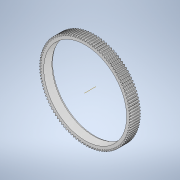
# Autodesk Inventor part: МТ10-3.00.00.01
Saved by Autodesk Inventor 2021 (Build 250183000, 183)
## iProperties
Created: 2022-06-08
Part Number: МТ10-3.00.00.01
Material: Типовые
Document SubType Name: Modeling
Designer: u
Density: 1 g/cm^3
Appearance: По умолчанию
Mass: 620.535 g
Surface Area: 1629.14 cm^2
Volume: 620.535 cm^3
Description: Колесо
Author: u
Title: Колесо
Autodesk Inventor part; units mm, degrees
ref_plane "YZ Plane" through (0, 0, 0) normal (1, 0, 0) x (0, 1, 0)
ref_plane "XZ Plane" through (0, 0, 0) normal (0, 1, 0) x (-1, 0, 0)
ref_plane "XY Plane" through (0, 0, 0) normal (0, 0, 1) x (1, 0, 0)
sketch "Эскиз1" plane through (0, 0, 0) normal (0, 0, 1) x (1, 0, 0)
  circle A0 centre (0, 0) radius 172
  circle A1 centre (0, 0) radius 189.5
  circle A2 centre (0, 0) radius 175.25
  dimension "d0" = 344
  dimension "d1" = 350.5
  dimension "d2" = 379
  constraints: 3 centre point, 3 coincident
  measures "d0" diameter of A0
  measures "d1" diameter of A2
  measures "d2" diameter of A1
extrude "Выдавливание1" add sketch "Эскиз1" along normal blind 40 contours A1 | A2
sketch "Эскиз3" plane through (0, 0, 0) normal (0, 0, -1) x (-1, 0, 0)
  circle A0 centre (0, 0) radius 183
  line L0 (-3.8538, 189.4608) -> (-1.5, 182.9939)
  line L1 (3.8538, 189.4608) -> (1.5, 182.9939)
  circle A1 centre (0, 0) radius 189.5 projected
  line L2 (0, 183) -> (0, 189.5)
  line L3 (-14.6636, 188.9318) -> (-11.9445, 182.6098)
  line L4 (-6.9686, 189.3718) -> (-8.9493, 182.781)
  line L5 (-25.4256, 187.7866) -> (-22.3499, 181.6301)
  line L6 (-17.7682, 188.6652) -> (-19.3695, 181.972)
  line L7 (-36.1046, 186.0288) -> (-32.6825, 180.0579)
  line L8 (-28.5099, 187.3431) -> (-29.7265, 180.5695)
  line L9 (-46.6659, 183.6642) -> (-42.9085, 177.8984)
  line L10 (-39.1586, 185.41) -> (-39.9865, 178.5779)
  line L11 (-57.075, 180.7006) -> (-52.9946, 175.1587)
  line L12 (-49.6796, 182.8721) -> (-50.1161, 176.0039)
  line L13 (-67.2979, 177.1475) -> (-62.9077, 171.8477)
  line L14 (-60.0385, 179.7377) -> (-60.0822, 172.8558)
  line L15 (-77.3012, 173.0167) -> (-72.6157, 167.9761)
  line L16 (-70.2016, 176.017) -> (-69.8524, 169.1439)
  line L17 (-87.0525, 168.3215) -> (-82.0868, 163.5566)
  line L18 (-80.1357, 171.7222) -> (-79.3947, 164.8802)
  line L19 (-96.5198, 163.0772) -> (-91.2902, 158.6036)
  line L20 (-89.8085, 166.8673) -> (-88.678, 160.0788)
  line L21 (-105.6723, 157.3011) -> (-100.1958, 153.1333)
  line L22 (-99.1882, 161.4681) -> (-97.6721, 154.7552)
  line L23 (-114.48, 151.0118) -> (-108.7746, 147.1635)
  line L24 (-108.2445, 155.5422) -> (-106.3476, 148.9268)
  line L25 (-122.9144, 144.23) -> (-116.9986, 140.7136)
  line L26 (-116.9477, 149.109) -> (-114.6762, 142.6127)
  line L27 (-130.9479, 136.9777) -> (-124.841, 133.8048)
  line L28 (-125.2694, 142.1894) -> (-122.6307, 135.8334)
  line L29 (-138.5542, 129.2787) -> (-132.2761, 126.4596)
  line L30 (-133.1825, 134.806) -> (-130.1853, 128.611)
  line L31 (-145.7086, 121.158) -> (-139.2798, 118.7019)
  line L32 (-140.6612, 126.9829) -> (-137.3152, 120.9691)
  line L33 (-152.3877, 112.642) -> (-145.8292, 110.557)
  line L34 (-147.6811, 118.7457) -> (-143.9973, 112.9327)
  line L35 (-158.5698, 103.7587) -> (-151.9029, 102.0514)
  line L36 (-154.2193, 110.1211) -> (-150.2096, 104.5278)
  line L37 (-164.2347, 94.5369) -> (-157.4812, 93.213)
  line L38 (-160.2545, 101.1373) -> (-155.932, 95.7821)
  line L39 (-169.3638, 85.0068) -> (-162.5458, 84.0706)
  line L40 (-165.7669, 91.8236) -> (-161.1458, 86.7239)
  line L41 (-173.9405, 75.1993) -> (-167.0802, 74.6539)
  line L42 (-170.7387, 82.2104) -> (-165.8339, 77.3828)
  line L43 (-177.9499, 65.1466) -> (-171.0696, 64.9938)
  line L44 (-175.1535, 72.329) -> (-169.9812, 67.7894)
  line L45 (-181.3788, 54.8814) -> (-174.501, 55.1216)
  line L46 (-178.9971, 62.2118) -> (-173.574, 57.9748)
  line L47 (-184.2161, 44.4372) -> (-177.3633, 45.0697)
  line L48 (-182.2567, 51.8916) -> (-176.6006, 47.9711)
  line L49 (-186.4526, 33.8481) -> (-179.647, 34.8707)
  line L50 (-184.9219, 41.4021) -> (-179.0512, 37.811)
  line L51 (-188.0808, 23.1485) -> (-181.3447, 24.558)
  line L52 (-186.9839, 30.7776) -> (-180.9178, 27.5275)
  line L53 (-189.0956, 12.3735) -> (-182.4509, 14.1652)
  line L54 (-188.436, 20.0528) -> (-182.1942, 17.1542)
  line L55 (-189.4936, 1.558) -> (-182.9621, 3.7262)
  line L56 (-189.2735, 9.2625) -> (-182.8764, 6.725)
  line L57 (-189.2735, -9.2625) -> (-182.8764, -6.725)
  line L58 (-189.4936, -1.558) -> (-182.9621, -3.7262)
  line L59 (-188.436, -20.0528) -> (-182.1942, -17.1542)
  line L60 (-189.0956, -12.3735) -> (-182.4509, -14.1652)
  line L61 (-186.9839, -30.7776) -> (-180.9178, -27.5275)
  line L62 (-188.0808, -23.1485) -> (-181.3447, -24.558)
  line L63 (-184.9219, -41.4021) -> (-179.0512, -37.811)
  line L64 (-186.4526, -33.8481) -> (-179.647, -34.8707)
  line L65 (-182.2567, -51.8916) -> (-176.6006, -47.9711)
  line L66 (-184.2161, -44.4372) -> (-177.3633, -45.0697)
  line L67 (-178.9971, -62.2118) -> (-173.574, -57.9748)
  line L68 (-181.3788, -54.8814) -> (-174.501, -55.1216)
  line L69 (-175.1535, -72.329) -> (-169.9812, -67.7894)
  line L70 (-177.9499, -65.1466) -> (-171.0696, -64.9938)
  line L71 (-170.7387, -82.2104) -> (-165.8339, -77.3828)
  line L72 (-173.9405, -75.1993) -> (-167.0802, -74.6539)
  line L73 (-165.7669, -91.8236) -> (-161.1458, -86.7239)
  line L74 (-169.3638, -85.0068) -> (-162.5458, -84.0706)
  line L75 (-160.2545, -101.1373) -> (-155.932, -95.7821)
  line L76 (-164.2347, -94.5369) -> (-157.4812, -93.213)
  line L77 (-154.2193, -110.1211) -> (-150.2096, -104.5278)
  line L78 (-158.5698, -103.7587) -> (-151.9029, -102.0514)
  line L79 (-147.6811, -118.7457) -> (-143.9973, -112.9327)
  line L80 (-152.3877, -112.642) -> (-145.8292, -110.557)
  line L81 (-140.6612, -126.9829) -> (-137.3152, -120.9691)
  line L82 (-145.7086, -121.158) -> (-139.2798, -118.7019)
  line L83 (-133.1825, -134.806) -> (-130.1853, -128.611)
  line L84 (-138.5542, -129.2787) -> (-132.2761, -126.4596)
  line L85 (-125.2694, -142.1894) -> (-122.6307, -135.8334)
  line L86 (-130.9479, -136.9777) -> (-124.841, -133.8048)
  line L87 (-116.9477, -149.109) -> (-114.6762, -142.6127)
  line L88 (-122.9144, -144.23) -> (-116.9986, -140.7136)
  line L89 (-108.2445, -155.5422) -> (-106.3476, -148.9268)
  line L90 (-114.48, -151.0118) -> (-108.7746, -147.1635)
  line L91 (-99.1882, -161.4681) -> (-97.6721, -154.7552)
  line L92 (-105.6723, -157.3011) -> (-100.1958, -153.1333)
  line L93 (-89.8085, -166.8673) -> (-88.678, -160.0788)
  line L94 (-96.5198, -163.0772) -> (-91.2902, -158.6036)
  line L95 (-80.1357, -171.7222) -> (-79.3947, -164.8802)
  line L96 (-87.0525, -168.3215) -> (-82.0868, -163.5566)
  line L97 (-70.2016, -176.017) -> (-69.8524, -169.1439)
  line L98 (-77.3012, -173.0167) -> (-72.6157, -167.9761)
  line L99 (-60.0385, -179.7377) -> (-60.0822, -172.8558)
  line L100 (-67.2979, -177.1475) -> (-62.9077, -171.8477)
  line L101 (-49.6796, -182.8721) -> (-50.1161, -176.0039)
  line L102 (-57.075, -180.7006) -> (-52.9946, -175.1587)
  line L103 (-39.1586, -185.41) -> (-39.9865, -178.5779)
  line L104 (-46.6659, -183.6642) -> (-42.9085, -177.8984)
  line L105 (-28.5099, -187.3431) -> (-29.7265, -180.5695)
  line L106 (-36.1046, -186.0288) -> (-32.6825, -180.0579)
  line L107 (-17.7682, -188.6652) -> (-19.3695, -181.972)
  line L108 (-25.4256, -187.7866) -> (-22.3499, -181.6301)
  line L109 (-6.9686, -189.3718) -> (-8.9493, -182.781)
  line L110 (-14.6636, -188.9318) -> (-11.9445, -182.6098)
  line L111 (3.8538, -189.4608) -> (1.5, -182.9939)
  line L112 (-3.8538, -189.4608) -> (-1.5, -182.9939)
  line L113 (14.6636, -188.9318) -> (11.9445, -182.6098)
  line L114 (6.9686, -189.3718) -> (8.9493, -182.781)
  line L115 (25.4256, -187.7866) -> (22.3499, -181.6301)
  line L116 (17.7682, -188.6652) -> (19.3695, -181.972)
  line L117 (36.1046, -186.0288) -> (32.6825, -180.0579)
  line L118 (28.5099, -187.3431) -> (29.7265, -180.5695)
  line L119 (46.6659, -183.6642) -> (42.9085, -177.8984)
  line L120 (39.1586, -185.41) -> (39.9865, -178.5779)
  line L121 (57.075, -180.7006) -> (52.9946, -175.1587)
  line L122 (49.6796, -182.8721) -> (50.1161, -176.0039)
  line L123 (67.2979, -177.1475) -> (62.9077, -171.8477)
  line L124 (60.0385, -179.7377) -> (60.0822, -172.8558)
  line L125 (77.3012, -173.0167) -> (72.6157, -167.9761)
  line L126 (70.2016, -176.017) -> (69.8524, -169.1439)
  line L127 (87.0525, -168.3215) -> (82.0868, -163.5566)
  line L128 (80.1357, -171.7222) -> (79.3947, -164.8802)
  line L129 (96.5198, -163.0772) -> (91.2902, -158.6036)
  line L130 (89.8085, -166.8673) -> (88.678, -160.0788)
  line L131 (105.6723, -157.3011) -> (100.1958, -153.1333)
  line L132 (99.1882, -161.4681) -> (97.6721, -154.7552)
  line L133 (114.48, -151.0118) -> (108.7746, -147.1635)
  line L134 (108.2445, -155.5422) -> (106.3476, -148.9268)
  line L135 (122.9144, -144.23) -> (116.9986, -140.7136)
  line L136 (116.9477, -149.109) -> (114.6762, -142.6127)
  line L137 (130.9479, -136.9777) -> (124.841, -133.8048)
  line L138 (125.2694, -142.1894) -> (122.6307, -135.8334)
  line L139 (138.5542, -129.2787) -> (132.2761, -126.4596)
  line L140 (133.1825, -134.806) -> (130.1853, -128.611)
  line L141 (145.7086, -121.158) -> (139.2798, -118.7019)
  line L142 (140.6612, -126.9829) -> (137.3152, -120.9691)
  line L143 (152.3877, -112.642) -> (145.8292, -110.557)
  line L144 (147.6811, -118.7457) -> (143.9973, -112.9327)
  line L145 (158.5698, -103.7587) -> (151.9029, -102.0514)
  line L146 (154.2193, -110.1211) -> (150.2096, -104.5278)
  line L147 (164.2347, -94.5369) -> (157.4812, -93.213)
  line L148 (160.2545, -101.1373) -> (155.932, -95.7821)
  line L149 (169.3638, -85.0068) -> (162.5458, -84.0706)
  line L150 (165.7669, -91.8236) -> (161.1458, -86.7239)
  line L151 (173.9405, -75.1993) -> (167.0802, -74.6539)
  line L152 (170.7387, -82.2104) -> (165.8339, -77.3828)
  line L153 (177.9499, -65.1466) -> (171.0696, -64.9938)
  line L154 (175.1535, -72.329) -> (169.9812, -67.7894)
  line L155 (181.3788, -54.8814) -> (174.501, -55.1216)
  line L156 (178.9971, -62.2118) -> (173.574, -57.9748)
  line L157 (184.2161, -44.4372) -> (177.3633, -45.0697)
  line L158 (182.2567, -51.8916) -> (176.6006, -47.9711)
  line L159 (186.4526, -33.8481) -> (179.647, -34.8707)
  line L160 (184.9219, -41.4021) -> (179.0512, -37.811)
  line L161 (188.0808, -23.1485) -> (181.3447, -24.558)
  line L162 (186.9839, -30.7776) -> (180.9178, -27.5275)
  line L163 (189.0956, -12.3735) -> (182.4509, -14.1652)
  line L164 (188.436, -20.0528) -> (182.1942, -17.1542)
  line L165 (189.4936, -1.558) -> (182.9621, -3.7262)
  line L166 (189.2735, -9.2625) -> (182.8764, -6.725)
  line L167 (189.2735, 9.2625) -> (182.8764, 6.725)
  line L168 (189.4936, 1.558) -> (182.9621, 3.7262)
  line L169 (188.436, 20.0528) -> (182.1942, 17.1542)
  line L170 (189.0956, 12.3735) -> (182.4509, 14.1652)
  line L171 (186.9839, 30.7776) -> (180.9178, 27.5275)
  line L172 (188.0808, 23.1485) -> (181.3447, 24.558)
  line L173 (184.9219, 41.4021) -> (179.0512, 37.811)
  line L174 (186.4526, 33.8481) -> (179.647, 34.8707)
  line L175 (182.2567, 51.8916) -> (176.6006, 47.9711)
  line L176 (184.2161, 44.4372) -> (177.3633, 45.0697)
  line L177 (178.9971, 62.2118) -> (173.574, 57.9748)
  line L178 (181.3788, 54.8814) -> (174.501, 55.1216)
  line L179 (175.1535, 72.329) -> (169.9812, 67.7894)
  line L180 (177.9499, 65.1466) -> (171.0696, 64.9938)
  line L181 (170.7387, 82.2104) -> (165.8339, 77.3828)
  line L182 (173.9405, 75.1993) -> (167.0802, 74.6539)
  line L183 (165.7669, 91.8236) -> (161.1458, 86.7239)
  line L184 (169.3638, 85.0068) -> (162.5458, 84.0706)
  line L185 (160.2545, 101.1373) -> (155.932, 95.7821)
  line L186 (164.2347, 94.5369) -> (157.4812, 93.213)
  line L187 (154.2193, 110.1211) -> (150.2096, 104.5278)
  line L188 (158.5698, 103.7587) -> (151.9029, 102.0514)
  line L189 (147.6811, 118.7457) -> (143.9973, 112.9327)
  line L190 (152.3877, 112.642) -> (145.8292, 110.557)
  line L191 (140.6612, 126.9829) -> (137.3152, 120.9691)
  line L192 (145.7086, 121.158) -> (139.2798, 118.7019)
  line L193 (133.1825, 134.806) -> (130.1853, 128.611)
  line L194 (138.5542, 129.2787) -> (132.2761, 126.4596)
  line L195 (125.2694, 142.1894) -> (122.6307, 135.8334)
  line L196 (130.9479, 136.9777) -> (124.841, 133.8048)
  line L197 (116.9477, 149.109) -> (114.6762, 142.6127)
  line L198 (122.9144, 144.23) -> (116.9986, 140.7136)
  line L199 (108.2445, 155.5422) -> (106.3476, 148.9268)
  line L200 (114.48, 151.0118) -> (108.7746, 147.1635)
  line L201 (99.1882, 161.4681) -> (97.6721, 154.7552)
  line L202 (105.6723, 157.3011) -> (100.1958, 153.1333)
  line L203 (89.8085, 166.8673) -> (88.678, 160.0788)
  line L204 (96.5198, 163.0772) -> (91.2902, 158.6036)
  line L205 (80.1357, 171.7222) -> (79.3947, 164.8802)
  line L206 (87.0525, 168.3215) -> (82.0868, 163.5566)
  line L207 (70.2016, 176.017) -> (69.8524, 169.1439)
  line L208 (77.3012, 173.0167) -> (72.6157, 167.9761)
  line L209 (60.0385, 179.7377) -> (60.0822, 172.8558)
  line L210 (67.2979, 177.1475) -> (62.9077, 171.8477)
  line L211 (49.6796, 182.8721) -> (50.1161, 176.0039)
  line L212 (57.075, 180.7006) -> (52.9946, 175.1587)
  line L213 (39.1586, 185.41) -> (39.9865, 178.5779)
  line L214 (46.6659, 183.6642) -> (42.9085, 177.8984)
  line L215 (28.5099, 187.3431) -> (29.7265, 180.5695)
  line L216 (36.1046, 186.0288) -> (32.6825, 180.0579)
  line L217 (17.7682, 188.6652) -> (19.3695, 181.972)
  line L218 (25.4256, 187.7866) -> (22.3499, 181.6301)
  line L219 (6.9686, 189.3718) -> (8.9493, 182.781)
  line L220 (14.6636, 188.9318) -> (11.9445, 182.6098)
  dimension "d18" = 366
  dimension "d19" = 1.5
  dimension "d20" = 3
  dimension "d21" = 20
  dimension "d24" = 360
  constraints: 442 end point, 6 point on circle, 1 centre point, 1 coincident, 1 equal length, 1 vertical, 1 vertical alignment, 661 other
  measures "d18" diameter of A0
  measures "d19" distance of L0.end L2.start
  measures "d20" distance of L1.end L0.end
  measures "d21" angle of L2 L0
extrude "Выдавливание3" cut sketch "Эскиз3" against normal through all contours A0 L195 A1 L196
extrude "Выдавливание2" cut sketch "Эскиз1" along normal blind 6 contours A2
pattern_circular "Круговой массив1" count 110 over 360 about axis through (0, 0, 0) along (0, 0, 1) of "Выдавливание3"
equation "\"d20\" = 2 * d19"
